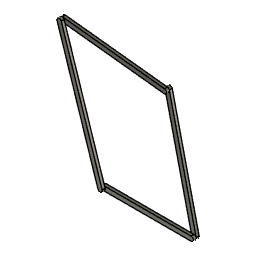
4_Bar_Link v1 (Autodesk Fusion 360 design; units mm, degrees)
Autodesk Fusion 360 part; units mm, degrees
sketch "Sketch5" plane through (0, 0, 0) normal (0, 1, 0) x (1, 0, 0)
  line L0 (0, -1.5) -> (60, -1.5)
  arc A0 (60, -1.5) -> (60, 1.5) centre (60, 0) ccw
  line L1 (60, 1.5) -> (0, 1.5)
  arc A1 (0, 1.5) -> (0, -1.5) centre (0, 0) ccw
  line L2 (0, 0) -> (60, 0) construction
  arc A2 (0, -12.5) -> (0, -15.5) centre (0, -14) ccw
  line L3 (0, -14) -> (90, -14) construction
  line L4 (90, -12.5) -> (0, -12.5)
  line L5 (0, -15.5) -> (90, -15.5)
  arc A3 (90, -15.5) -> (90, -12.5) centre (90, -14) ccw
  arc A4 (80, -45.5) -> (80, -42.5) centre (80, -44) ccw
  arc A5 (70, -31.5) -> (70, -28.5) centre (70, -30) ccw
  line L6 (0, -31.5) -> (70, -31.5)
  line L7 (0, -45.5) -> (80, -45.5)
  line L8 (0, -30) -> (70, -30) construction
  line L9 (0, -44) -> (80, -44) construction
  arc A6 (0, -28.5) -> (0, -31.5) centre (0, -30) ccw
  line L10 (80, -42.5) -> (0, -42.5)
  line L11 (70, -28.5) -> (0, -28.5)
  arc A7 (0, -42.5) -> (0, -45.5) centre (0, -44) ccw
  dimension "d1" = 3
  dimension "d2" = 60
  dimension "d3" = 3
  dimension "d4" = 90
  dimension "d5" = 3
  dimension "d6" = 70
  dimension "d7" = 3
  dimension "d8" = 80
  constraint tangent L0 A0
  constraint tangent A0 L1
  constraint parallel L0 L1
  constraint tangent L1 A1
  constraint tangent L0 A1
  constraint horizontal L2
  constraint coincident A1.centre L2.start
  constraint tangent L5 A3
  constraint tangent L4 A3
  constraint parallel L4 L5
  constraint tangent A2 L4
  constraint tangent A2 L5
  constraint horizontal L3
  constraint tangent A5 L6
  constraint tangent A5 L11
  constraint parallel L6 L11
  constraint tangent A6 L11
  constraint tangent L6 A6
  constraint horizontal L8
  constraint tangent A4 L7
  constraint tangent A4 L10
  constraint parallel L7 L10
  constraint tangent L10 A7
  constraint tangent L7 A7
  constraint horizontal L9
  measures "d1" diameter of A0
  measures "d2" distance of A1.centre A0.centre
  measures "d3" diameter of A3
  measures "d4" distance of A2.centre L3.end
  measures "d5" diameter of A5
  measures "d6" distance of L8.start A5.centre
  measures "d7" diameter of A4
  measures "d8" distance of L9.start A4.centre
extrude "Extrude1" add sketch "Sketch5" along normal blind 2 makes body 1 at (30, 0, 13.5) makes body 2 at (53.3333, 0, 44.5) makes body 3 at (40, 0, 0.5) makes body 4 at (23.3333, 0, 30.5)
copy_body "Body->Comp1" bodies 1 removing the originals makes body 5 in component "Component"
copy_body "Body->Comp2" bodies 2 removing the originals makes body 6 in component "Component'"
copy_body "Body->Comp3" bodies 3 removing the originals makes body 7 in component "Component''"
copy_body "Body->Comp4" bodies 4 removing the originals makes body 8 in component "Component'''"
sketch "Sketch1" plane through (0, 0, 0) normal (0, 1, 0) x (1, 0, 0)
  line L0 (0, 0) -> (28, 0)
  constraint coincident L0.start origin
  constraint horizontal L0
sketch "Sketch2" plane through (0, 0, 0) normal (0, 1, 0) x (1, 0, 0)
  line L0 (28, 0) -> (42, -21)
sketch "Sketch3" plane through (0, 0, 0) normal (0, 1, 0) x (1, 0, 0)
  line L0 (42, -21) -> (-21, -21)
  constraint horizontal L0
sketch "Sketch4" plane through (0, 0, 0) normal (0, 1, 0) x (1, 0, 0)
  line L0 (-23, -21) -> (0, 0)
  constraint coincident L0.end origin
component "Component" placed x (-0.794145, 0, -0.607728) y (0, -1, 0) z (-0.607728, 0, 0.794145) at (79.9812, 0, 43.5775)
component "Component'" placed x (0.731585, 0, -0.68175) y (0, 1, 0) z (0.68175, 0, 0.731585) at (-28.5238, 2, 22.3503)
component "Component''" placed x (1, 0, 0) y (0, 1, 0) z (0, 0, 1) at (0, 0, 0)
component "Component'''" placed x (0.999998, 0, 0.002222) y (0, 1, 0) z (-0.002222, 0, 0.999998) at (1.5399, 0, 24.5401)
